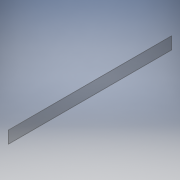
# Autodesk Inventor part: Bumper Support Plate
Saved by Autodesk Inventor 2019.4 (Build 234330000, 330)
## iProperties
Created: 2019-12-14
Part Number: Bumper Support Plate
Material: Polycarbonate, Smoke
Document SubType Name: Modeling
Designer: admin
Density: 1.2 g/cm^3
Appearance: Polycarbonate - Smoked
Author: admin
Autodesk Inventor part; units mm, degrees
ref_plane "YZ Plane" through (0, 0, 0) normal (1, 0, 0) x (0, 1, 0)
ref_plane "XZ Plane" through (0, 0, 0) normal (0, 1, 0) x (-1, 0, 0)
ref_plane "XY Plane" through (0, 0, 0) normal (0, 0, 1) x (1, 0, 0)
sketch "Sketch1" plane through (0, 0, 0) normal (1, 0, 0) x (0, 1, 0)
  line L0 (0, 0) -> (60, 0)
  line L1 (60, 0) -> (60, -800)
  line L2 (60, -800) -> (0, -800)
  line L3 (0, -800) -> (0, 0)
  dimension "d0" = 800
  dimension "d1" = 60
  constraints: 8 end point, 2 parallel, 1 horizontal, 1 perpendicular
  measures "d0" distance of L0.end L1.end
  measures "d1" distance of L0.start L0.end
extrude "Extrusion1" add sketch "Sketch1" along normal blind 2
body "Solid1"
